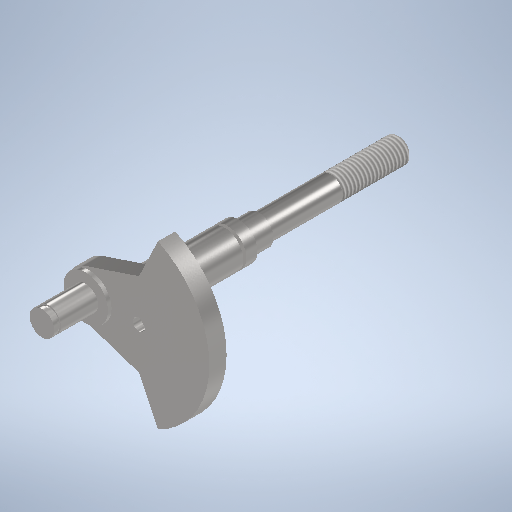
# Autodesk Inventor part: Welle
Saved by Autodesk Inventor 2025 (Build 290162010, 162A)
## iProperties
Created: 2024-04-30
Part Number: Welle
Material: Stahl, galvanisiert
Document SubType Name: Modeling
Designer: ffogue
Density: 7.85 g/cm^3
Appearance: Galvanisiert
Author: ffogue
Autodesk Inventor part; units mm, degrees
ref_plane "YZ Plane" through (0, 0, 0) normal (1, 0, 0) x (0, 1, 0)
sketch "Skizze1" plane through (0, 0, 0) normal (0, 1, 0) x (-1, 0, 0)
  line L0 (0, 16.9269) -> (22.2468, 9.4832)
  arc A0 (22.2468, -9.4832) -> (22.2468, 9.4832) centre (19.0737, 0) ccw
  line L1 (22.2468, -9.4832) -> (0, -16.9269)
  line L2 (0, 0) -> (24.8397, 0) construction
  line L3 (0, 16.9269) -> (-7.6399, 32.9444)
  arc A1 (-7.6399, 32.9444) -> (-7.6399, -32.9444) centre (8.0737, 0) ccw
  line L4 (-7.6399, -32.9444) -> (0, -16.9269)
  dimension "d0" = 37
  dimension "d2" = 129
  dimension "d3" = 36.5
  dimension "d5" = 10
  dimension "d53" = 11
  constraints: 10 end point, 4 point on circle, 3 symmetric about line, 2 centre point, 2 vertical alignment, 1 horizontal, 1 horizontal alignment, 1 point on line, 1 tangent
  measures "d0" angle of L1 L0
  measures "d2" angle of L4 L3
  measures "d3" radius of A1
  measures "d5" radius of A0
  measures "d53" distance of A1.centre A0.centre
extrude "Extrusion1" add sketch "Skizze1" along normal mid plane 7
ref_plane "Arbeitsebene1" through (0, 0, 0) normal (0, 0, 1) x (1, 0, 0)
sketch "Skizze5" plane through (0, 0, 0) normal (0, 0, 1) x (1, 0, 0)
  line L0 (-22.2468, -3.5) -> (0, -3.5) projected
  line L1 (-29.0737, -3.5) -> (-22.2468, -3.5) projected
  line L2 (-29.0737, -3.5) -> (-29.0737, 3.5) projected
  line L3 (-29.0737, -3.5) -> (-29.0737, -5)
  line L4 (-29.0737, -5) -> (-25.0737, -5)
  line L5 (-25.0737, -5) -> (-25.0737, -20)
  line L6 (-25.0737, -20) -> (-24.5737, -20)
  line L7 (-24.5737, -20) -> (-24.5737, -21.1)
  line L8 (-24.5737, -21.1) -> (-25.0737, -21.1)
  line L9 (-25.0737, -21.1) -> (-25.0737, -22.7)
  line L10 (-25.0737, -22.7) -> (-20.0737, -22.7)
  line L11 (-20.0737, -22.7) -> (-20.0737, -3.5)
  point P0 (0, 0)
  point P1 (-24.8237, -20)
  dimension "d32" = 9
  dimension "d33" = 1.5
  dimension "d35" = 1.1
  dimension "d36" = 15
  dimension "d37" = 10
  dimension "d38" = 9
  dimension "d39" = 18
  dimension "d41" = 2.7
  constraints: 18 end point, 7 perpendicular, 3 point on line, 1 midpoint, 1 vertical
  measures "d32" distance between parallel lines of L11 L2
  measures "d33" distance between parallel lines of L1 L4
  measures "d35" distance between parallel lines of L6 L8
  measures "d36" distance from line of point (-24.824, -20) L4
  measures "d37" diameter of L5 L11
  measures "d38" diameter of L7 L11
  measures "d39" diameter of L3 L11
  measures "d41" distance from line of L10 point (-24.824, -20)
revolve "Umdrehung2" add sketch "Skizze5" angle 360 about axis through (-20.0737, -22.7, 0) along (0, 1, 0)
sketch "Skizze3" plane through (0, 0, 0) normal (0, 0, 1) x (1, 0, 0)
  line L0 (0, 3.5) -> (-22.2468, 3.5) projected
  line L1 (-22.2468, 3.5) -> (-29.0737, 3.5) projected
  line L2 (-29.0737, -3.5) -> (-29.0737, 3.5) projected
  line L3 (-20.0737, 5) -> (-17.5737, 5)
  line L4 (-17.5737, 5) -> (-17.5737, 18)
  line L5 (-17.5737, 18) -> (-16.5737, 18)
  line L6 (-16.5737, 18) -> (-16.5737, 40.3)
  line L7 (-16.5737, 40.3) -> (-14.0737, 40.3)
  line L8 (-14.0737, 40.3) -> (-14.0737, 41.5)
  line L9 (-14.0737, 41.5) -> (-16.5737, 41.5)
  line L10 (-16.5737, 41.5) -> (-16.5737, 46)
  line L11 (-16.5737, 46) -> (-15.0737, 46)
  line L12 (-15.0737, 46) -> (-15.0737, 54)
  line L13 (-15.0737, 54) -> (-14.0737, 54)
  line L14 (-14.0737, 54) -> (-14.0737, 111)
  line L15 (-14.0737, 111) -> (-9.0737, 111)
  line L16 (-9.0737, 111) -> (-9.0737, 3.5)
  line L17 (-20.0737, 5) -> (-20.0737, 3.5)
  line L18 (-11.0737, -5) -> (-29.0737, -5) construction
  line L19 (-11.0737, -5) -> (-11.0737, -3.5) construction
  line L20 (-29.0737, -5) -> (-29.0737, -3.5) construction
  line L21 (-25.0737, -20) -> (-25.0737, -5) construction
  line L22 (-15.0737, -20) -> (-15.0737, -5) construction
  line L23 (-15.0737, -22.7) -> (-25.0737, -22.7) construction
  point P0 (-15.8237, 46)
  point P1 (-9.0737, 3.5)
  point P2 (-20.0737, -5)
  dimension "d13" = 10
  dimension "d14" = 12
  dimension "d15" = 15
  dimension "d16" = 17
  dimension "d18" = 22
  dimension "d20" = 1.5
  dimension "d21" = 1.2
  dimension "d22" = 4.5
  dimension "d44" = 13
  dimension "d45" = 8
  dimension "d46" = 57
  dimension "d47" = 28
  dimension "d48" = 106
  constraints: 30 end point, 11 perpendicular, 6 point on line, 2 midpoint, 1 vertical, 1 vertical alignment
  measures "d13" diameter of L14 L16
  measures "d14" diameter of L12 L16
  measures "d15" diameter of L10 L16
  measures "d16" diameter of L4 L16
  measures "d18" diameter of L17 L16
  measures "d20" distance of L3.start L17.end
  measures "d21" distance between parallel lines of L9 L7
  measures "d22" distance from line of point (-15.824, 46) L9
  measures "d44" distance of L3.end L4.end
  measures "d45" distance between parallel lines of L13 L11
  measures "d46" distance of L13.end L14.end
  measures "d47" distance from line of point (-15.824, 46) L5
  measures "d48" distance between parallel lines of L15 L3
revolve "Umdrehung1" add sketch "Skizze3" angle 360 about axis through (-9.0737, 111, 0) along (0, -1, 0)
thread "Gewinde1" size "M10x1.5" class "6g" standard "ISO Metric profile" length 28
chamfer "Fasen1" distance 1 angle 45 1 edges at (-4.0737, 111, 0)
ref_plane "Work Plane3" through (0, 0, 8.5) normal (0, 0, 1) x (1, 0, 0)
sketch "Sketch8" plane through (-8.0737, -3.5, 0) normal (0, -1, 0) x (1, 0, 0)
  circle A0 centre (8.0737, 0) radius 2.5
  dimension "d54" = 5
  constraints: 1 centre point, 1 coincident
  measures "d54" diameter of A0
extrude "Extrusion2" cut sketch "Sketch8" against normal blind 3
